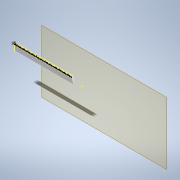
# Autodesk Inventor part: liniau
Saved by Autodesk Inventor 2021 (Build 250183000, 183)
## iProperties
Created: 2021-06-18
Part Number: liniau
Material: Ogólny
Document SubType Name: Modeling
Designer: Wojciech Wołczek
Density: 1 g/cm^3
Appearance: Domyślna
Author: Wojciech Wołczek
Autodesk Inventor part; units mm, degrees
ref_plane "YZ Plane" through (0, 0, 0) normal (1, 0, 0) x (0, 1, 0)
ref_plane "XZ Plane" through (0, 0, 0) normal (0, 1, 0) x (-1, 0, 0)
ref_plane "XY Plane" through (0, 0, 0) normal (0, 0, 1) x (1, 0, 0)
ref_plane "Płaszczyzna konstrukcyjna1" through (0, 0, 0) normal (0, 0, 1) x (1, 0, 0)
sketch "Szkic1" plane through (0, 0, 0) normal (0, 0, 1) x (1, 0, 0)
  line L0 (-468.6039, 25) -> (-68.6039, 25)
  line L1 (-68.6039, 25) -> (-68.6039, -25)
  line L2 (-68.6039, -25) -> (-468.6039, -25)
  line L3 (-468.6039, -25) -> (-468.6039, 25)
  line L4 (-468.6039, 25) -> (-68.6039, -25) construction
  line L5 (-68.6039, 25) -> (-468.6039, -25) construction
  point P0 (0, 0)
  point P1 (-268.6039, 0)
  dimension "d0" = 400
  dimension "d1" = 50
  constraints: 12 end point, 2 midpoint, 2 parallel, 1 horizontal, 1 perpendicular
  measures "d0" distance of L1.end L2.end
  measures "d1" distance of L0.end L1.end
extrude "Wyciągnięcie proste1" add sketch "Szkic1" along normal blind 10
chamfer "Faza1" distance 34 distance2 7 1 edges at (-268.6039, -25, 10) measured on face at (-268.6039, -24.5, 10)
sketch "Szkic2" plane through (0, 0, 10) normal (0, 0, 1) x (1, 0, 0)
  line L0 (-68.6039, 25) -> (-468.6039, 25) projected
  line L1 (-468.6039, 25) -> (-468.6039, 15)
  line L2 (-468.6039, 25) -> (-468.6039, -25) projected
  line L3 (-463.6039, 25) -> (-463.6039, 15)
  line L4 (-458.6039, 25) -> (-458.6039, 15)
  line L5 (-453.6039, 25) -> (-453.6039, 15)
  line L6 (-448.6039, 25) -> (-448.6039, 15)
  line L7 (-443.6039, 25) -> (-443.6039, 15)
  line L8 (-438.6039, 25) -> (-438.6039, 15)
  line L9 (-433.6039, 25) -> (-433.6039, 15)
  line L10 (-428.6039, 25) -> (-428.6039, 15)
  line L11 (-423.6039, 25) -> (-423.6039, 15)
  line L12 (-418.6039, 25) -> (-418.6039, 15)
  line L13 (-413.6039, 25) -> (-413.6039, 15)
  line L14 (-408.6039, 25) -> (-408.6039, 15)
  line L15 (-403.6039, 25) -> (-403.6039, 15)
  line L16 (-398.6039, 25) -> (-398.6039, 15)
  line L17 (-393.6039, 25) -> (-393.6039, 15)
  line L18 (-388.6039, 25) -> (-388.6039, 15)
  line L19 (-383.6039, 25) -> (-383.6039, 15)
  line L20 (-378.6039, 25) -> (-378.6039, 15)
  line L21 (-373.6039, 25) -> (-373.6039, 15)
  line L22 (-368.6039, 25) -> (-368.6039, 15)
  line L23 (-363.6039, 25) -> (-363.6039, 15)
  line L24 (-358.6039, 25) -> (-358.6039, 15)
  line L25 (-353.6039, 25) -> (-353.6039, 15)
  line L26 (-348.6039, 25) -> (-348.6039, 15)
  line L27 (-343.6039, 25) -> (-343.6039, 15)
  line L28 (-338.6039, 25) -> (-338.6039, 15)
  line L29 (-333.6039, 25) -> (-333.6039, 15)
  line L30 (-328.6039, 25) -> (-328.6039, 15)
  line L31 (-323.6039, 25) -> (-323.6039, 15)
  line L32 (-318.6039, 25) -> (-318.6039, 15)
  line L33 (-313.6039, 25) -> (-313.6039, 15)
  line L34 (-308.6039, 25) -> (-308.6039, 15)
  line L35 (-303.6039, 25) -> (-303.6039, 15)
  line L36 (-298.6039, 25) -> (-298.6039, 15)
  line L37 (-293.6039, 25) -> (-293.6039, 15)
  line L38 (-288.6039, 25) -> (-288.6039, 15)
  line L39 (-283.6039, 25) -> (-283.6039, 15)
  line L40 (-278.6039, 25) -> (-278.6039, 15)
  line L41 (-273.6039, 25) -> (-273.6039, 15)
  line L42 (-268.6039, 25) -> (-268.6039, 15)
  line L43 (-263.6039, 25) -> (-263.6039, 15)
  line L44 (-258.6039, 25) -> (-258.6039, 15)
  line L45 (-253.6039, 25) -> (-253.6039, 15)
  line L46 (-248.6039, 25) -> (-248.6039, 15)
  line L47 (-243.6039, 25) -> (-243.6039, 15)
  line L48 (-238.6039, 25) -> (-238.6039, 15)
  line L49 (-233.6039, 25) -> (-233.6039, 15)
  line L50 (-228.6039, 25) -> (-228.6039, 15)
  line L51 (-223.6039, 25) -> (-223.6039, 15)
  line L52 (-218.6039, 25) -> (-218.6039, 15)
  line L53 (-213.6039, 25) -> (-213.6039, 15)
  line L54 (-208.6039, 25) -> (-208.6039, 15)
  line L55 (-203.6039, 25) -> (-203.6039, 15)
  line L56 (-198.6039, 25) -> (-198.6039, 15)
  line L57 (-193.6039, 25) -> (-193.6039, 15)
  line L58 (-188.6039, 25) -> (-188.6039, 15)
  line L59 (-183.6039, 25) -> (-183.6039, 15)
  line L60 (-178.6039, 25) -> (-178.6039, 15)
  line L61 (-173.6039, 25) -> (-173.6039, 15)
  line L62 (-168.6039, 25) -> (-168.6039, 15)
  line L63 (-163.6039, 25) -> (-163.6039, 15)
  line L64 (-158.6039, 25) -> (-158.6039, 15)
  line L65 (-153.6039, 25) -> (-153.6039, 15)
  line L66 (-148.6039, 25) -> (-148.6039, 15)
  line L67 (-143.6039, 25) -> (-143.6039, 15)
  line L68 (-138.6039, 25) -> (-138.6039, 15)
  line L69 (-133.6039, 25) -> (-133.6039, 15)
  line L70 (-128.6039, 25) -> (-128.6039, 15)
  line L71 (-123.6039, 25) -> (-123.6039, 15)
  line L72 (-118.6039, 25) -> (-118.6039, 15)
  line L73 (-113.6039, 25) -> (-113.6039, 15)
  line L74 (-108.6039, 25) -> (-108.6039, 15)
  line L75 (-103.6039, 25) -> (-103.6039, 15)
  line L76 (-98.6039, 25) -> (-98.6039, 15)
  line L77 (-93.6039, 25) -> (-93.6039, 15)
  line L78 (-88.6039, 25) -> (-88.6039, 15)
  line L79 (-83.6039, 25) -> (-83.6039, 15)
  line L80 (-78.6039, 25) -> (-78.6039, 15)
  line L81 (-73.6039, 25) -> (-73.6039, 15)
  point P0 (0, 0)
  dimension "d7" = 10
  dimension "d10" = 5
  constraints: 160 end point, 1 horizontal, 1 point on line, 237 other
  measures "d7" distance of L0.end L1.end
  measures "d10" distance of L0.end L3.start
sketch "Szkic3" plane through (0, 0, 10) normal (0, 0, 1) x (1, 0, 0)
  line L0 (-73.6039, 25) -> (-73.6039, 15) projected
  line L1 (-118.6039, 25) -> (-118.6039, 15) projected
  line L2 (-113.6039, 25) -> (-113.6039, 15) projected
  line L3 (-68.6039, 25) -> (-468.6039, 25) projected
  line L4 (-74.1039, 5) -> (-73.1039, 5)
  line L5 (-73.1039, 5) -> (-73.1039, 25)
  line L6 (-73.1039, 25) -> (-74.1039, 25)
  line L7 (-74.1039, 25) -> (-74.1039, 5)
  line L8 (-74.1039, 5) -> (-73.1039, 25) construction
  line L9 (-73.1039, 5) -> (-74.1039, 25) construction
  point P0 (0, 0)
  dimension "d15" = 1
  constraints: 12 end point, 2 midpoint, 2 parallel, 1 horizontal, 1 perpendicular, 1 point on line
  measures "d15" distance of L6.end L5.end
extrude "Wyciągnięcie proste2" cut sketch "Szkic3" against normal blind 1
pattern_linear "Szyk prostokątny1" count 80 spacing 5 along (-1, 0, 0) of "Wyciągnięcie proste2"
